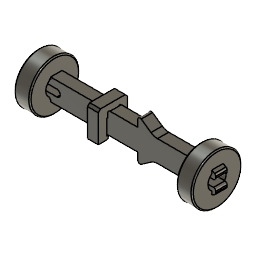
_Low Fidelity Shaft.0cec9413-75b8-48d4-a7a7-27a8910e8c9c (Autodesk Fusion 360 design; units mm, degrees)
Autodesk Fusion 360 part; units mm, degrees
sketch "Sketch1" plane through (0, 0, 0) normal (0, 1, 0) x (1, 0, 0)
  line L0 (0, 0) -> (0, -3.75) construction
  line L1 (0, -3.75) -> (7.5, -3.75)
  line L2 (0, -3.75) -> (0, -4.75)
  line L3 (0, -4.75) -> (-1.7321, -3.75)
  line L4 (0, -4.75) -> (1.5486, -4.75) construction
  line L5 (-1.7321, -3.75) -> (-1.7321, 0)
  line L6 (7.5, -3.75) -> (7.5, -4.75)
  line L7 (7.5, -4.75) -> (64.65, -4.75)
  line L8 (-1.7321, 0) -> (36.075, 0) construction
  line L9 (36.075, 0) -> (36.075, -4.75) construction
  line L10 (73.8821, -3.75) -> (73.8821, 0)
  line L11 (72.15, -4.75) -> (73.8821, -3.75)
  line L12 (72.15, -3.75) -> (64.65, -3.75)
  line L13 (72.15, -3.75) -> (72.15, -4.75)
  line L14 (64.65, -3.75) -> (64.65, -4.75)
  line L15 (64.65, -4.75) -> (7.5, -4.75)
  line L16 (73.8821, 3.75) -> (73.8821, 0)
  line L17 (72.15, 4.75) -> (73.8821, 3.75)
  line L18 (72.15, 3.75) -> (64.65, 3.75)
  line L19 (72.15, 3.75) -> (72.15, 4.75)
  line L20 (64.65, 3.75) -> (64.65, 4.75)
  line L21 (64.65, 4.75) -> (7.5, 4.75)
  line L22 (7.5, 3.75) -> (7.5, 4.75)
  line L23 (0, 3.75) -> (7.5, 3.75)
  line L24 (0, 3.75) -> (0, 4.75)
  line L25 (0, 4.75) -> (-1.7321, 3.75)
  line L26 (-1.7321, 3.75) -> (-1.7321, 0)
  line L27 (-1.7321, 0) -> (73.8821, 0)
  point P0 (36.075, -4.75)
  dimension "d1" = 3.75
  dimension "d2" = 7.5
  dimension "d4" = 150
  dimension "d5" = 57.15
  dimension "d8" = 4.75
  constraint coincident L0.start origin
  constraint vertical L0
  constraint perpendicular L0 L1
  constraint perpendicular L1 L2
  constraint horizontal L4
  constraint coincident L1 L3.end
  constraint vertical L5
  constraint perpendicular L4 L6
  constraint perpendicular L6 L7
  constraint horizontal L0.start L5.end
  constraint perpendicular L5 L8
  constraint horizontal L2.end L6.end
  constraint midpoint L7 P0
  constraint vertical L8.end P0
  constraint coincident P0 L9.end
  constraint symmetric L0.end L9 L12.start
  constraint symmetric L1.end L9 L12.end
  constraint symmetric L2.end L9 L11.start
  constraint symmetric L3.end L9 L10.start
  constraint symmetric L5.end L9 L10.end
  constraint symmetric L6.end L9 L7.end
  constraint symmetric L7.end L9 L6.end
  constraint symmetric L0.end L8 L23.start
  constraint symmetric L1.end L8 L22.start
  constraint symmetric L2.end L8 L24.end
  constraint symmetric L3.end L8 L25.end
  constraint symmetric L5.end L8 L26.end
  constraint symmetric L6.end L8 L21.end
  constraint symmetric L8 L10.start L16.start
  constraint symmetric L8 L10.end L16.end
  constraint symmetric L8 L11.start L17.start
  constraint symmetric L8 L12.start L18.start
  constraint symmetric L8 L12.end L18.end
  constraint symmetric L8 L7.end L20.end
  constraint symmetric L8 L6.end L21.end
  measures "d1" distance of L0.start L0.end
  measures "d2" distance of L0.end L1.end
  measures "d4" angle of L3 L4
  measures "d5" distance of L6.end L7.end
  measures "d8" distance of L8 L15
extrude "Extrude1" add sketch "Sketch1" along normal blind 5 makes body 1
sketch "Sketch2" plane through (0, 5, 0) normal (0, 1, 0) x (-1, 0, 0)
  line L0 (0, -3.75) -> (0, -4.75)
  line L1 (0, -4.75) -> (1.7321, -3.75)
  line L2 (1.7321, -3.75) -> (1.7321, 3.75)
  line L3 (1.7321, 3.75) -> (0, 4.75)
  line L4 (0, 4.75) -> (0, 3.75)
  line L5 (0, 3.75) -> (-7.5, 3.75)
  line L6 (-7.5, 3.75) -> (-7.5, 4.75)
  line L7 (-7.5, 4.75) -> (-64.65, 4.75)
  line L8 (-64.65, 4.75) -> (-64.65, 3.75)
  line L9 (-64.65, 3.75) -> (-72.15, 3.75)
  line L10 (-72.15, 3.75) -> (-72.15, 4.75)
  line L11 (-72.15, 4.75) -> (-73.8821, 3.75)
  line L12 (-73.8821, 3.75) -> (-73.8821, -3.75)
  line L13 (-73.8821, -3.75) -> (-72.15, -4.75)
  line L14 (-72.15, -4.75) -> (-72.15, -3.75)
  line L15 (-72.15, -3.75) -> (-64.65, -3.75)
  line L16 (-64.65, -3.75) -> (-64.65, -4.75)
  line L17 (-64.65, -4.75) -> (-7.5, -4.75)
  line L18 (-7.5, -4.75) -> (-7.5, -3.75)
  line L19 (-7.5, -3.75) -> (0, -3.75)
  line L20 (-73.8821, 0) -> (1.7321, 0) construction
  line L21 (-36.075, 4.75) -> (-36.075, -4.75) construction
  line L22 (1.7321, 1.5) -> (-10.2679, 1.5)
  arc A0 (-10.2679, 1.5) -> (-10.2679, -1.5) centre (-10.2679, 0) ccw
  line L23 (-10.2679, -1.5) -> (1.7321, -1.5)
  arc A1 (1.7321, -1.5) -> (1.7321, 1.5) centre (1.7321, 0) ccw
  line L24 (1.7321, 0) -> (-10.2679, 0) construction
  line L25 (-61.8821, -1.5) -> (-73.8821, -1.5)
  arc A2 (-61.8821, -1.5) -> (-61.8821, 1.5) centre (-61.8821, 0) ccw
  line L26 (-73.8821, 1.5) -> (-61.8821, 1.5)
  arc A3 (-73.8821, 1.5) -> (-73.8821, -1.5) centre (-73.8821, 0) ccw
  dimension "d9" = 1.5
  dimension "d10" = 12
  constraint midpoint L12 L20.start
  constraint midpoint L2 L20.end
  constraint midpoint L7 L21.start
  constraint midpoint L17 L21.end
  constraint tangent L22 A0
  constraint tangent A0 L23
  constraint parallel L22 L23
  constraint tangent L23 A1
  constraint tangent L22 A1
  constraint coincident L20 A0.centre
  constraint perpendicular L2 L24
  constraint coincident L20.end A1.centre
  constraint symmetric L21 L22.start L26.start
  constraint symmetric L21 L22.end A2.end
  constraint symmetric L21 A0.end L25.start
  constraint symmetric L21 L23.end L25.end
  constraint symmetric L21 A0 A2
  constraint symmetric L21 A1 A3
  measures "d9" radius of A1
  measures "d10" distance of L2 A0.centre
extrude "Extrude2" cut sketch "Sketch2" against normal through all contours L2 L22 A0 L23 | L12 L25 A2 L26 bodies 1
sketch "Sketch3" plane through (0, 0, 0) normal (0, -1, 0) x (1, 0, 0)
  line L0 (61.8821, 1.5) -> (73.8821, 1.5)
  line L1 (73.8821, 1.5) -> (73.8821, 3.75)
  line L2 (73.8821, 3.75) -> (72.15, 4.75)
  line L3 (72.15, 4.75) -> (72.15, 3.75)
  line L4 (72.15, 3.75) -> (64.65, 3.75)
  line L5 (64.65, 3.75) -> (64.65, 4.75)
  line L6 (64.65, 4.75) -> (7.5, 4.75)
  line L7 (7.5, 4.75) -> (7.5, 3.75)
  line L8 (7.5, 3.75) -> (0, 3.75)
  line L9 (0, 3.75) -> (0, 4.75)
  line L10 (0, 4.75) -> (-1.7321, 3.75)
  line L11 (-1.7321, 3.75) -> (-1.7321, 1.5)
  line L12 (-1.7321, 1.5) -> (10.2679, 1.5)
  arc A0 (10.2679, -1.5) -> (10.2679, 1.5) centre (10.2679, 0) ccw
  line L13 (10.2679, -1.5) -> (-1.7321, -1.5)
  line L14 (-1.7321, -1.5) -> (-1.7321, -3.75)
  line L15 (-1.7321, -3.75) -> (0, -4.75)
  line L16 (0, -4.75) -> (0, -3.75)
  line L17 (0, -3.75) -> (7.5, -3.75)
  line L18 (7.5, -3.75) -> (7.5, -4.75)
  line L19 (7.5, -4.75) -> (64.65, -4.75)
  line L20 (64.65, -4.75) -> (64.65, -3.75)
  line L21 (64.65, -3.75) -> (72.15, -3.75)
  line L22 (72.15, -3.75) -> (72.15, -4.75)
  line L23 (72.15, -4.75) -> (73.8821, -3.75)
  line L24 (73.8821, -3.75) -> (73.8821, -1.5)
  line L25 (73.8821, -1.5) -> (61.8821, -1.5)
  arc A1 (61.8821, 1.5) -> (61.8821, -1.5) centre (61.8821, 0) ccw
  line L26 (36.075, 4.75) -> (36.075, -4.75) construction
  line L27 (32.65, 4.75) -> (32.65, -4.75) construction
  line L28 (39.5, 4.75) -> (39.5, -4.75) construction
  line L29 (39.5, 4.75) -> (39.5, 9.75)
  line L30 (39.5, 9.75) -> (46.6407, 4.75)
  line L31 (32.65, 0) -> (39.5, 0) construction
  line L32 (39.5, -4.75) -> (39.5, -9.75)
  line L33 (39.5, -9.75) -> (46.6407, -4.75)
  line L34 (32.65, 4.75) -> (27.65, 4.75)
  line L35 (27.65, 4.75) -> (27.65, 1.75)
  line L36 (27.65, 1.75) -> (32.65, 1.75)
  line L37 (32.65, 1.75) -> (32.65, 4.75)
  line L38 (32.65, 1.75) -> (32.65, -2.25)
  line L39 (32.65, -2.25) -> (27.65, -2.25) construction
  line L40 (27.65, -2.25) -> (27.65, -1.15)
  line L41 (27.65, -1.15) -> (32.65, -1.15)
  line L42 (27.65, -2.25) -> (27.65, -3.35)
  line L43 (27.65, -3.35) -> (32.65, -3.35)
  line L44 (32.65, -2.25) -> (32.65, -3.35)
  dimension "d13" = 6.85
  dimension "d14" = 35
  dimension "d15" = 5
  dimension "d16" = 5
  dimension "d17" = 3
  dimension "d44" = 1.1
  dimension "d45" = 1.1
  dimension "d46" = 4
  constraint midpoint L6 L26.start
  constraint midpoint L19 L26.end
  constraint coincident L6 L27.start
  constraint coincident L19 L27.end
  constraint perpendicular L19 L27
  constraint coincident L6 L28.start
  constraint coincident L19 L28.end
  constraint perpendicular L19 L28
  constraint symmetric L26 L27 L28
  constraint perpendicular L6 L29
  constraint coincident L6 L30.end
  constraint midpoint L27 L31.start
  constraint midpoint L28 L31.end
  constraint symmetric L28.start L31 L28.end
  constraint symmetric L29.end L31 L32.end
  constraint symmetric L30.end L31 L33.end
  constraint horizontal L34
  constraint vertical L35
  constraint horizontal L36
  constraint vertical L37
  constraint coincident L27 L38.end
  constraint perpendicular L35 L39
  constraint perpendicular L39 L40
  constraint perpendicular L27 L41
  constraint coincident L27 L41.end
  constraint perpendicular L39 L42
  constraint coincident L27 L43.end
  constraint perpendicular L27 L43
  measures "d13" distance of L27 L28
  measures "d14" angle of L6 L30
  measures "d15" distance of L28.start L29.end
  measures "d16" distance of L27.start L34.end
  measures "d17" distance of L27.start L36.end
  measures "d44" distance of L39.end L40.end
  measures "d45" distance of L39.end L42.end
  measures "d46" distance of L36.end L38.end
extrude "Extrude3" add sketch "Sketch3" against normal blind 5 contours L6 L29 L30 | L19 L32 L33 bodies 1
extrude "Extrude4" cut sketch "Sketch3" against normal blind 5 contours L6 L34 L35 L36 L37 bodies 1
fillet "Fillet1" radius 1 2 edges at (39.5, 2.5, 9.75) (39.5, 2.5, -9.75) on bodies 1
fillet "Fillet1" radius 5 2 edges at (46.6407, 2.5, 4.75) (46.6407, 2.5, -4.75) on bodies 1
fillet "Fillet1" radius 1 8 edges at (73.8821, 2.5, 3.75) (73.8821, 2.5, 1.5) (73.8821, 2.5, -1.5) (73.8821, 2.5, -3.75) (-1.7321, 2.5, 3.75) (-1.7321, 2.5, 1.5) (-1.7321, 2.5, -1.5) (-1.7321, 2.5, -3.75) on bodies 1
fillet "Fillet1" radius 1 2 edges at (32.65, 2.5, 4.75) (27.65, 2.5, 4.75) on bodies 1
sketch "Sketch1 (2)" plane through (32.65, 0, 0) normal (-1, 0, 0) x (0, -1, 0) in component "Collar"
  line L0 (-5, 3.75) -> (-5, 1.75)
  line L1 (-5, 1.75) -> (0, 1.75)
  line L2 (0, 1.75) -> (0, 3.75)
  line L3 (0, 1.75) -> (-5, 1.75)
  line L4 (-5, 1.75) -> (0, 1.75)
  line L5 (0.25, 1.75) -> (-5.1734, 1.75)
  line L6 (-7.9234, 6.75) -> (3, 6.75)
  line L7 (4, 5.75) -> (4, -6.5)
  line L8 (-8.9234, -6.5) -> (-8.9234, 5.75)
  line L9 (0.25, -6.5) -> (4, -6.5)
  line L10 (-5.2669, -6.5) -> (-8.9234, -6.5)
  line L11 (3, 6.75) -> (4, 5.75)
  line L12 (-7.9234, 6.75) -> (-8.9234, 5.75)
  arc A0 (0.25, -5) -> (0.25, -6.5) centre (0.25, -5.75) ccw
  line L13 (0.25, 1.75) -> (0.25, -5)
  arc A1 (-5.2669, -6.5) -> (-5.1734, -5.0058) centre (-5.2669, -5.75) ccw
  line L14 (-5.1734, -5.0058) -> (-5.1734, 1.75)
  point P0 (-8.9234, 6.75)
  point P1 (4, 6.75)
  dimension "d38" = 1
  dimension "d39" = 1
  dimension "d40" = 1
  dimension "d41" = 1
  dimension "d42" = 1.5
  dimension "d43" = 1.5
  dimension "d50" = 7.5
  dimension "d52" = 3.75
  dimension "d54" = 5
  dimension "d55" = 3.75
  constraint horizontal L5
  constraint horizontal L6
  constraint vertical L7
  constraint vertical L8
  constraint perpendicular L7 L9
  constraint perpendicular L8 L10
  constraint coincident P1 L6
  constraint coincident P1 L7
  constraint coincident P0 L6
  constraint coincident P0 L8
  constraint coincident L9.start L13
  constraint coincident A0.centre L13
  constraint coincident L0.end L5
  constraint equal L7 L8
  constraint horizontal A0.centre A1.centre
  constraint coincident L10.start A1.start
  measures "d38" distance of P1 L6.end
  measures "d39" distance of P1 L7.start
  measures "d40" distance of P0 L6.start
  measures "d41" distance of P0 L8.end
  measures "d42" diameter of A0
  measures "d43" diameter of A1
  measures "d50" distance of L5 A1.centre
  measures "d52" distance of L7 L13
  measures "d54" distance of L5 L6
  measures "d55" distance of L8 L14
extrude "Extrude1'" add sketch "Sketch1 (2)" along normal blind 4.75 separate body makes body 2 in component "Collar"
copy_body "Body->Comp1" bodies 1 removing the originals makes body 3 in component "Snap Axis"
move_face "MoveFace1" to x (1, 0, 0) y (0, 1, 0) z (0, 0, 1) at (-6.35, 0, 0) 23 faces at (32.65, 1.6667, 2.4167) (32.9263, 1.6667, 4.4401) (29.3167, 1.6667, 1.75) (27.65, 3.3333, 2.4167) (27.1082, 1.6667, 4.6388) (7.5, 1.6667, 4.0833) (2.5, 1.6667, 3.75) (0, 1.6667, 4.0833) (-0.4107, 1.6667, 4.5129) (-1.3158, 1.6667, 3.9846) (-1.7321, 1.6667, 2.9484) (-0.7796, 3.3333, 1.5011) (2.9346, 3.3333, 1.5) (10.4173, 1.6667, -1.4925) (7.5, 1.6667, -4.0833) (2.5, 1.6667, -3.75) (6.6013, 3.3333, -1.5) (-1.7309, 3.3333, -2.4524) (-1.7321, 1.6667, -2.9484) (-1.2746, 1.6667, -4.0127) (-0.4107, 1.6667, -4.5129) (0, 1.6667, -4.0833) (13.8833, 1.6667, 4.75) on bodies 3 in component "Snap Axis"
other "GeometricRelationship1"
ref_plane "WorkPlane1" through (39.25, 2.6734, -2.8363) normal (1, 0, 0) x (0, 0, -1)
ref_plane "WorkPlane2" through (78.4821, 2.6734, 2.8363) normal (1, 0, 0) x (0, 0, -1)
sketch "Sketch4" plane through (78.4821, 0, 0) normal (1, 0, 0) x (0, 0, -1)
  circle A0 centre (0, 2.5) radius 11
  circle A1 centre (0, 2.5) radius 4
  dimension "d63" = 22
  dimension "d64" = 8
  constraint concentric A0 A1
  measures "d63" diameter of A0
  measures "d64" diameter of A1
extrude "Extrude1''" add sketch "Sketch4" against normal blind 7 sketch seen with x (1, 0, 0) y (0, 1, 0) z (0, 0, 1) at (-6.35, -0.1734, 0) bodies 3 in component "Snap Axis"
fillet "Fillet1'" radius 0.5 2 edges at (65.1321, 6.3044, 10.2556) (72.1321, -1.6512, 10.2556) on bodies 3 in component "Snap Axis"
mirror "Mirror1" about plane through (32.9, 2.5, -2.8363) normal (1, 0, 0) of "Extrude1''", "Fillet1'" in component "Snap Axis"
sketch "Sketch5" plane through (32.65, 0, 0) normal (-1, 0, 0) x (0, -1, 0)
sketch "Sketch6" plane through (32.65, 0, 0) normal (-1, 0, 0) x (0, -1, 0)
  line L0 (-0.1734, 3.75) -> (-5.1734, 3.75)
  line L1 (-5.1734, 3.75) -> (-5.1734, 1.75)
  line L2 (-5.1734, 1.75) -> (-0.1734, 1.75)
  line L3 (-0.1734, 1.75) -> (-0.1734, 3.75)
  arc A0 (0.25, -5) -> (0.25, -6.5) centre (0.25, -5.75) ccw
  line L4 (0.25, 1.75) -> (0.25, -5)
  line L5 (-8.9234, -6.5) -> (-8.9234, 5.75)
  line L6 (-5.2669, -6.5) -> (-8.9234, -6.5)
  line L7 (0.25, -6.5) -> (4, -6.5)
  line L8 (0.25, 1.75) -> (-5.1734, 1.75)
  line L9 (-7.9234, 6.75) -> (3, 6.75)
  line L10 (-5, 1.75) -> (0, 1.75)
  line L11 (-7.9234, 6.75) -> (-8.9234, 5.75)
  line L12 (0, 1.75) -> (0, 3.75)
  line L13 (-5, 1.75) -> (0, 1.75)
  line L14 (-5, 3.75) -> (-5, 1.75)
  line L15 (3, 6.75) -> (4, 5.75)
  line L16 (-5.1734, -5.0058) -> (-5.1734, 1.75)
  line L17 (0, 1.75) -> (-5, 1.75)
  line L18 (4, 5.75) -> (4, -6.5)
  arc A1 (-5.2669, -6.5) -> (-5.1734, -5.0058) centre (-5.2669, -5.75) ccw
  point P0 (-8.9234, 6.75)
  point P1 (4, 6.75)
  dimension "d71" = 1
  dimension "d72" = 1
  dimension "d73" = 1
  dimension "d74" = 1
  dimension "d75" = 1.5
  dimension "d76" = 1.5
  dimension "d77" = 7.5
  dimension "d78" = 3.75
  dimension "d79" = 5
  dimension "d80" = 3.75
  constraint horizontal L8
  constraint horizontal L9
  constraint vertical L18
  constraint vertical L5
  constraint perpendicular L7 L18
  constraint perpendicular L5 L6
  constraint coincident P1 L9
  constraint coincident P1 L18
  constraint coincident P0 L9
  constraint coincident P0 L5
  constraint coincident A0.end L4
  constraint coincident A0.centre L4
  constraint coincident L10.start L8
  constraint equal L5 L18
  constraint horizontal A0.centre A1.centre
  constraint coincident L6.start A1.start
  measures "d71" distance of L9.end P1
  measures "d72" distance of L15.end P1
  measures "d73" distance of L9.start P0
  measures "d74" distance of L5.end P0
  measures "d75" diameter of A0
  measures "d76" diameter of A1
  measures "d77" distance of A1.centre L8
  measures "d78" distance of L4 L18
  measures "d79" distance of L8 L9
  measures "d80" distance of L5 L16
component "Collar" placed x (1, 0, 0) y (0, 1, 0) z (0, 0, 1) at (0, 0, 0)
component "Snap Axis" placed x (1, 0, 0) y (0, 1, 0) z (0, 0, 1) at (6.35, 0.1734, 0)
equation "d13 = 6.35 mm + 0.5 mm"
equation "d39 = d38"
equation "d41 = d40"
equation "d72 = d38"
equation "d74 = d40"
